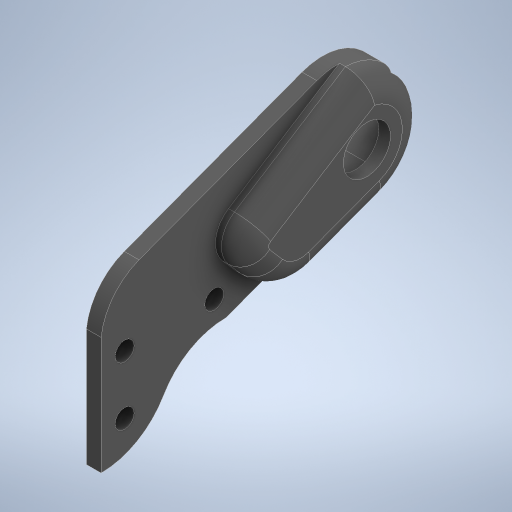
# Autodesk Inventor part: fore_arm_side_right
Saved by Autodesk Inventor 2024.1 (Build 281209000, 209)
## iProperties
Created: 2025-01-27
Part Number: fore_arm_side_right
Material: 一般
Document SubType Name: Modeling
Designer: hibik
Density: 1 g/cm^3
Appearance: 既定
Author: hibik
Autodesk Inventor part; units mm, degrees
ref_plane "YZ Plane" through (0, 0, 0) normal (1, 0, 0) x (0, 1, 0)
ref_plane "XZ Plane" through (0, 0, 0) normal (0, 1, 0) x (-1, 0, 0)
ref_plane "XY Plane" through (0, 0, 0) normal (0, 0, 1) x (1, 0, 0)
sketch "スケッチ1" plane through (0, 0, 0) normal (0, 1, 0) x (-1, 0, 0)
  line L0 (11.25, 0) -> (-11.25, 0)
  line L1 (-11.25, 0) -> (-11.25, -120)
  line L2 (-11.25, -120) -> (11.25, -120)
  line L3 (11.25, -120) -> (11.25, 0)
  point P0 (0, 0)
  point P1 (0, 0)
  dimension "d0" = 22.5
  dimension "d3" = 120
  constraints: 8 end point, 2 parallel, 1 coincident, 1 horizontal, 1 midpoint, 1 perpendicular
  measures "d0" distance of L0.start L0.end
  measures "d3" distance of L2.end L0.start
extrude "押し出し1" add sketch "スケッチ1" along normal blind 2
sketch "スケッチ2" plane through (0, 0, 0) normal (0, -1, 0) x (1, 0, 0)
  line L0 (19, -120) -> (-19, -120)
  line L1 (-19, -120) -> (-19, -103.05)
  line L2 (-19, -103.05) -> (19, -103.05)
  line L3 (19, -103.05) -> (19, -120)
  line L4 (11.25, -120) -> (-11.25, -120) projected
  point P0 (0, 0)
  point P1 (0, -120)
  dimension "d6" = 38
  dimension "d11" = 16.95
  constraints: 8 end point, 2 midpoint, 2 parallel, 1 collinear, 1 horizontal, 1 perpendicular
  measures "d6" distance of L0.start L0.end
  measures "d11" distance of L0.end L1.end
extrude "押し出し2" add sketch "スケッチ2" against normal blind 13.44
sketch "スケッチ4" plane through (11.25, 0, -103.05) normal (0, 0, 1) x (1, 0, 0)
  circle A0 centre (-11.25, 20) radius 20
  line L0 (7.75, 0) -> (0, 0) projected
  line L1 (-22.5, 0) -> (0, 0) projected
  point P0 (-11.25, 0)
  point P1 (-11.25, 0)
  dimension "d12" = 40
  constraints: 1 centre point, 1 midpoint, 1 tangent, 1 vertical alignment
  measures "d12" diameter of A0
extrude "押し出し4" cut sketch "スケッチ4" along normal through all
sketch "スケッチ5" plane through (11.25, 0, -103.05) normal (0, 0, 1) x (1, 0, 0)
  circle A0 centre (-11.25, 20) radius 20
  arc A1 (-11.25, 0) -> (-2.5322, 2) centre (-11.25, 20) ccw projected
  line L0 (-30.25, 13.44) -> (7.75, 13.44)
  line L1 (7.75, 13.44) -> (7.75, -5)
  line L2 (7.75, -5) -> (-30.25, -5)
  line L3 (-30.25, -5) -> (-30.25, 13.44)
  line L4 (7.75, 0) -> (7.75, 13.44) projected
  line L5 (7.75, 0) -> (0, 0) projected
  line L6 (-30.25, 4.22) -> (-11.25, 20)
  line L7 (-11.25, 20) -> (7.75, 4.22)
  point P0 (3.875, 0)
  point P1 (7.6436, 13.44)
  point P2 (-30.1436, 13.44)
  point P3 (7.75, 4.22)
  point P4 (4.1356, 7.2218)
  point P5 (-26.6356, 7.2218)
  point P6 (-3.3514, 13.44)
  point P7 (-19.1486, 13.44)
  dimension "d15" = 5
  constraints: 12 end point, 3 midpoint, 2 concentric, 2 parallel, 1 centre point, 1 collinear, 1 horizontal, 1 horizontal alignment, 1 perpendicular, 1 point on line
  measures "d15" distance from line of L2 point (3.875, 0)
extrude "押し出し5" add sketch "スケッチ5" along normal up to surface (103.05 mm away) contours A0 L7 L1 L2 L3 L6
sketch "スケッチ24" plane through (11.25, 0, -103.05) normal (0, 0, -1) x (-1, 0, 0)
  line L0 (-7.75, 0) -> (11.25, 0) projected
  line L1 (-7.75, -5) -> (-7.75, 0) projected
  line L2 (30.25, -5) -> (-7.75, -5) projected
  line L3 (30.25, 0) -> (30.25, -5) projected
  line L4 (11.25, 0) -> (30.25, 0) projected
  point P0 (11.25, 0)
extrude "押し出し22" add sketch "スケッチ24" along normal up to surface (16.95 mm away)
sketch "スケッチ25" plane through (19, 13.44, -103.05) normal (1, 0, 0) x (0, 0, -1)
  line L0 (-103.05, -13.44) -> (-103.05, -6.2182) projected
  line L1 (16.95, -18.44) -> (16.95, 0) projected
  line L2 (16.95, -13.44) -> (-40.05, -13.44)
  line L3 (-40.05, -13.44) -> (-40.05, 1.46)
  line L4 (-40.05, 1.46) -> (16.95, 1.46)
  line L5 (16.95, 1.46) -> (16.95, -13.44)
  dimension "d77" = 14.9
  dimension "d78" = 57
  constraints: 8 end point, 2 parallel, 2 point on line, 1 horizontal, 1 perpendicular
  measures "d77" distance of L4.end L2.start
  measures "d78" distance of L3.end L4.end
extrude "押し出し23" add sketch "スケッチ25" against normal up to surface (38 mm away)
sketch "スケッチ26" plane through (19, -5, 0) normal (1, 0, 0) x (0, 0, -1)
  line L0 (63, 12.2218) -> (0, 12.2218) projected
  circle A0 centre (63, 12.2218) radius 12.2218
  line L1 (0, 0) -> (120, 0) projected
  circle A1 centre (84.1688, 0) radius 12.2218
  line L2 (84.1688, 12.2218) -> (120, 12.2218)
  line L3 (120, 0) -> (120, 19.9) projected
  point P0 (0, 5)
  point P1 (73.5844, 6.1109)
  point P2 (63, 0)
  constraints: 2 end point, 2 horizontal, 2 point on line, 1 centre point, 1 coincident, 1 tangent, 5 other
extrude "押し出し24" cut sketch "スケッチ26" against normal through all contours A1 L1 A0 | A1 L1 | L2 L3 L1 A1 picked at (80.2991, 4.512)
sketch "スケッチ28" plane through (19, -5, 0) normal (1, 0, 0) x (0, 0, -1)
  circle A0 centre (103.05, 29.95) radius 18.95
  line L0 (120, 12.2218) -> (120, 19.9) projected
  line L1 (120, 19.9) -> (63, 19.9) projected
  line L2 (84.1688, 12.2218) -> (120, 12.2218) projected
  point P0 (0, 5)
  point P1 (96.3557, 12.2218)
  point P2 (86.9845, 19.9)
  dimension "d83" = 16.95
  dimension "d84" = 10.05
  dimension "d85" = 37.9
  constraints: 1 centre point
  measures "d83" distance from line of L0 A0.centre
  measures "d84" distance from line of L1 A0.centre
  measures "d85" diameter of A0
extrude "押し出し25" cut sketch "スケッチ28" against normal through all contours L1 A0 L2 | L1 L0 L2 A0
fillet "フィレット4" radius 2 1 edges at (0, 7.2218, -96.3557)
ref_plane "作業平面4" through (22.5, -5, 0) normal (1, 0, 0) x (0, 0, -1)
ref_plane "作業平面5" through (-23.5, -5, 0) normal (-1, 0, 0) x (0, 0, 1)
sketch "スケッチ29" plane through (22.5, -5, 0) normal (1, 0, 0) x (0, 0, -1)
  line L0 (63, 19.9) -> (63, 9.22) projected
  line L1 (86.9845, 19.9) -> (63, 19.9) projected
  arc A0 (84.1688, 12.2218) -> (73.5844, 6.1109) centre (84.1688, 0) ccw projected
  arc A1 (63, 0) -> (73.5844, 6.1109) centre (63, 12.2218) ccw projected
  line L2 (63, 9.22) -> (0, 9.22) projected
  line L3 (63, 9.22) -> (63, -0.3745)
  line L4 (84.1688, 12.2218) -> (84.1688, 19.9)
  point P0 (0, 5)
  point P1 (63, 0)
  constraints: 4 end point, 1 perpendicular, 1 point on line, 1 vertical
extrude "押し出し26" add sketch "スケッチ29" against normal up to surface (46 mm away)
fillet "フィレット5" radius 2 4 edges at (19, 11.0609, -84.1688) (19, -0.39, -63) (-19, -0.39, -63) (-19, 11.0609, -84.1688)
ref_plane "作業平面6" through (0, 20, -45) normal (0, 0, 1) x (1, 0, 0)
sketch "スケッチ31" plane through (0, 20, -45) normal (0, 0, 1) x (1, 0, 0)
  circle A0 centre (0, 0) radius 22
  arc A1 (-15.3856, -12.7782) -> (15.3856, -12.7782) centre (0, 0) ccw projected
  point P0 (0, -20)
  dimension "d95" = 44
  constraints: 1 centre point, 1 concentric
  measures "d95" diameter of A0
extrude "押し出し27" cut sketch "スケッチ31" along normal blind 12
sketch "スケッチ32" plane through (22.5, -5, 0) normal (1, 0, 0) x (0, 0, -1)
  line L0 (63, 19.9) -> (63, 0) projected
  arc A0 (63, 0) -> (73.5844, 6.1109) centre (63, 12.2218) ccw projected
  arc A1 (84.1688, 12.2218) -> (73.5844, 6.1109) centre (84.1688, 0) ccw projected
  line L1 (84.1688, 12.2218) -> (84.1688, 19.9) projected
  line L2 (84.1688, 19.9) -> (63, 19.9) projected
  circle A2 centre (103.05, 29.95) radius 4
  circle A3 centre (103.05, 29.95) radius 10
  line L3 (99.5506, 39.3177) -> (106.5494, 20.5823)
  line L4 (106.5494, 20.5823) -> (68.1093, 6.2226)
  line L5 (68.1093, 6.2226) -> (61.1105, 24.9581)
  line L6 (61.1105, 24.9581) -> (99.5506, 39.3177)
  point P0 (0, 5)
  dimension "d98" = 40.05
  dimension "d99" = 10.05
  dimension "d100" = 8
  dimension "d101" = 20
  constraints: 8 end point, 2 centre point, 2 parallel, 2 point on circle, 2 point on line, 1 coincident, 1 midpoint, 1 perpendicular
  measures "d98" distance from line of A2.centre L0
  measures "d99" distance from line of L2 A2.centre
  measures "d100" diameter of A2
  measures "d101" diameter of A3
extrude "押し出し28" add sketch "スケッチ32" along normal blind 7.5 contours L5 L4 A1 A0 L0 | L5 L6 A3 L4 L1 L2 | L2 L1 A1 L4 L5 | L3 A2 A3 | A3 L3 A2
sketch "スケッチ33" plane through (22.5, -5, 0) normal (-1, 0, 0) x (0, 0, 1)
  line L0 (73.7681, 73.9475) -> (-168.83, 73.9475)
  line L1 (-168.83, 73.9475) -> (-168.83, -57.4645)
  line L2 (-168.83, -57.4645) -> (73.7681, -57.4645)
  line L3 (73.7681, -57.4645) -> (73.7681, 73.9475)
  point P0 (0, 5)
  constraints: 8 end point, 2 parallel, 1 horizontal, 1 perpendicular
extrude "押し出し29" cut sketch "スケッチ33" along normal through all
sketch "スケッチ35" plane through (22.5, -5, 0) normal (-1, 0, 0) x (0, 0, 1)
  circle A0 centre (-103.05, 29.95) radius 4 projected
  line L0 (-99.5506, 39.3177) -> (-61.1105, 24.9581) projected
  circle A1 centre (-103.05, 29.95) radius 6.25
  circle A2 centre (-87.1249, 24.001) radius 2.75
  line L1 (-103.05, 29.95) -> (-87.1249, 24.001)
  line L2 (-87.1249, 24.001) -> (-88.8308, 19.4342)
  line L3 (-85.6528, 26.3238) -> (-99.7043, 35.2291)
  line L4 (-103.9849, 23.7703) -> (-87.5362, 21.282)
  line L5 (-102.1151, 36.1297) -> (-109.8336, 37.2973)
  line L6 (-106.3957, 24.6709) -> (-112.9893, 28.8496)
  arc A3 (-99.5506, 39.3177) -> (-106.5494, 20.5823) centre (-103.05, 29.95) ccw projected
  line L7 (-103.05, 29.95) -> (-102.2758, 32.0226)
  point P0 (0, 5)
  point P1 (-88.0872, 21.4249)
  point P2 (-88.1083, 21.3685)
  dimension "d106" = 12.5
  dimension "d107" = 5.5
  dimension "d108" = 17
  constraints: 14 end point, 8 point on circle, 5 tangent, 2 centre point, 2 perpendicular, 1 coincident, 1 parallel, 2 other
  measures "d106" diameter of A1
  measures "d107" diameter of A2
  measures "d108" distance from line of A0.centre L2
extrude "押し出し30" cut sketch "スケッチ35" against normal blind 5.5 contours A0 | A1 | A1 L3 A2 L1 | L1 A2 L2 L4 A1 | A1 L6 A3 L5 | A2 L2 L1 | L1 L2 A2
sketch "スケッチ36" plane through (30, -5, 0) normal (1, 0, 0) x (0, 0, -1)
  circle A0 centre (67, 6) radius 1.6
  circle A1 centre (67, 15.9) radius 1.6
  circle A2 centre (82.1688, 15.9) radius 1.6
  line L0 (86.1688, 12.2218) -> (86.1688, 19.9) projected
  line L1 (84.1688, 19.9) -> (63, 19.9) projected
  line L2 (63, 19.9) -> (63, 0) projected
  point P0 (0, 5)
  dimension "d111" = 3.2
  dimension "d112" = 4
  dimension "d113" = 4
  dimension "d114" = 4
  dimension "d115" = 4
  dimension "d116" = 6
  constraints: 3 centre point, 2 equal radius, 1 vertical alignment
  measures "d111" diameter of A0
  measures "d112" distance from line of L0 A2.centre
  measures "d113" distance from line of L1 A2.centre
  measures "d114" distance from line of L1 A1.centre
  measures "d115" distance from line of L2 A1.centre
  measures "d116" vertical distance of L2.end A0.centre
extrude "押し出し31" cut sketch "スケッチ36" against normal through all
sketch "スケッチ37" plane through (22.5, -5, 0) normal (-1, 0, 0) x (0, 0, 1)
  line L0 (-84.1688, 19.9) -> (-63, 19.9) projected
  line L1 (-84.1688, 19.9) -> (-86.1688, 19.9) projected
  line L2 (-84.1688, 12.2218) -> (-84.1688, 19.9) projected
  arc A0 (-88.0872, 21.4249) -> (-85.6528, 26.3238) centre (-87.1249, 24.001) ccw projected
  line L3 (-99.7043, 35.2291) -> (-85.6528, 26.3238) projected
  line L4 (-88.1083, 21.3685) -> (-103.9849, 23.7703) projected
  line L5 (-99.5506, 39.3177) -> (-61.1105, 24.9581) projected
  line L6 (-106.5384, 41.9281) -> (-84.5822, 28.0132)
  arc A1 (-99.5506, 39.3177) -> (-109.8336, 37.2973) centre (-103.05, 29.95) ccw projected
  circle A2 centre (-87.1249, 24.001) radius 4.75
  line L7 (-61.1105, 24.9581) -> (-63, 19.9) projected
  point P0 (0, 5)
  point P1 (-103.4071, 39.9436)
  point P2 (-84.7282, 19.9)
  dimension "d119" = 2
  constraints: 2 end point, 1 coincident, 1 parallel, 1 point on line, 4 other
  measures "d119" distance between parallel lines of L3 L6
fillet "フィレット7" radius 10 1 edges at (26.25, 19.9581, -61.1105)
sketch "スケッチ38" plane through (30, -5, 0) normal (1, 0, 0) x (0, 0, -1)
  circle A0 centre (67, 15.9) radius 1.6 projected
  circle A1 centre (67, 6) radius 1.6 projected
  circle A2 centre (82.1688, 15.9) radius 1.6 projected
  circle A3 centre (67, 15.9) radius 3
  circle A4 centre (82.1688, 15.9) radius 3
  circle A5 centre (67, 6) radius 3
  point P0 (0, 5)
  dimension "d124" = 6
  dimension "d125" = 6
  dimension "d126" = 6
  constraints: 3 centre point, 2 coincident, 1 concentric
  measures "d124" diameter of A3
  measures "d125" diameter of A4
  measures "d126" diameter of A5
extrude "押し出し33" cut sketch "スケッチ38" against normal blind 5 contours A0 | A1 | A2 | A3 | A4 | A5
sketch "スケッチ39" plane through (30, -5, 0) normal (1, 0, 0) x (0, 0, -1)
  line L0 (106.5384, 41.9281) -> (84.5822, 28.0132) projected
  circle A0 centre (87.1249, 24.001) radius 4.75 projected
  line L1 (84.1688, 19.9) -> (63, 19.9) projected
  line L2 (83.5344, 20.8912) -> (89.3628, 14.1621)
  line L3 (84.1688, 12.2218) -> (106.5494, 20.5823) projected
  circle A1 centre (82.1688, 15.9) radius 3 projected
  circle A2 centre (67, 15.9) radius 3 projected
  circle A3 centre (82.1688, 15.9) radius 3 projected
  circle A4 centre (67, 6) radius 3 projected
  arc A5 (69.428, 28.0652) -> (63, 19.9) centre (72.9274, 18.6975) ccw projected
  line L4 (63, 19.9) -> (63, 0) projected
  arc A6 (63, 0) -> (73.5844, 6.1109) centre (63, 12.2218) ccw projected
  arc A7 (84.1688, 12.2218) -> (73.5844, 6.1109) centre (84.1688, 0) ccw projected
  line L5 (84.1688, 12.2218) -> (106.5494, 20.5823) projected
  arc A8 (106.5494, 20.5823) -> (99.5506, 39.3177) centre (103.05, 29.95) ccw projected
  line L6 (99.5506, 39.3177) -> (69.428, 28.0652) projected
  circle A9 centre (103.05, 29.95) radius 4 projected
  point P0 (0, 5)
  point P1 (103.4071, 39.9436)
  dimension "d129" = 4.3
  constraints: 2 end point, 1 point on circle, 1 point on line, 1 tangent
  measures "d129" distance from line of L2 A1.centre
extrude "押し出し34" cut sketch "スケッチ39" against normal up to surface (5 mm away) contours L0 A0 L2 L3 A7 A6 L4 A5 L6 A8
fillet "フィレット8" radius 8 1 edges at (27.5, 9.1621, -89.3628)
fillet "フィレット9" radius 4 6 edges at (30, 28.9784, -93.9947) (30, 19.6924, -82.4255) (30, 14.6275, -84.629) (30, 10.8497, -89.7933) (30, 13.3448, -100.5597) (30, 26.552, -112.9208)
equation "\"d113\" = d112"
equation "\"d114\" = d112"
equation "\"d115\" = d114"
